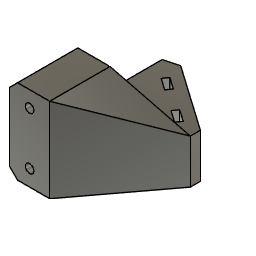
DirectDrive_SpoolHolder (Autodesk Fusion 360 design; units mm, degrees)
Autodesk Fusion 360 part; units mm, degrees
note: some values were not read from the file. Set by a fixed rule: which sketch regions a step uses.
sketch "Sketch1" plane through (0, 0, 0) normal (0, 0, 1) x (1, 0, 0) in component "Spool Holder"
  line L0 (10, 15) -> (-10, 15)
  line L1 (-10, 15) -> (-10, -15)
  line L2 (-10, -15) -> (10, -15)
  line L3 (10, -15) -> (10, 15)
  line L4 (10, 15) -> (-10, -15) construction
  line L5 (-10, 15) -> (10, -15) construction
  line L6 (10, 15) -> (50, 15)
  line L7 (50, 15) -> (50, 20)
  line L8 (50, 20) -> (17.2339, 42.9431)
  line L9 (50, 20) -> (46.0037, 20) construction
  line L10 (50, 15) -> (10, -15)
  line L11 (17.2339, 42.9431) -> (10, 32.612)
  line L12 (17.2339, 42.9431) -> (32.2339, 42.9431) construction
  line L13 (10, 15) -> (10, 32.612)
  line L14 (10, 32.612) -> (10, 41)
  line L15 (10, 41) -> (17.2339, 42.9431)
  dimension "d1" = 30
  dimension "d2" = 20
  dimension "d3" = 40
  dimension "d4" = 5
  dimension "d5" = 145
  dimension "d6" = 40
  dimension "d7" = 125
  constraint perpendicular L0 L1
  constraint parallel L0 L2
  constraint parallel L1 L3
  constraint horizontal L0
  constraint coincident L4 origin
  constraint coincident L5 origin
  constraint perpendicular L3 L6
  constraint perpendicular L6 L7
  constraint horizontal L9
  constraint horizontal L12
  constraint perpendicular L6 L13
  constraint vertical L14
  measures "d1" distance of L0.end L1.end
  measures "d2" distance of L1.end L2.end
  measures "d3" distance of L0.start L6.end
  measures "d4" distance of L6.end L7.end
  measures "d5" angle of L8 L9
  measures "d6" distance of L7.end L8.end
  measures "d7" angle of L11 L12
extrude "Extrude1" add sketch "Sketch1" along normal blind 42 in component "Spool Holder"
sketch "Sketch2" plane through (0, 0, 42) normal (0, 0, 1) x (-1, 0, 0) in component "Spool Holder"
  line L0 (10, -15) -> (10, 15)
  line L1 (10, 15) -> (-10, 15)
  line L2 (-10, 15) -> (-50, -15)
  line L3 (-50, -15) -> (-50, -20)
  line L4 (-50, -20) -> (-17.2339, -42.9431)
  line L5 (-10, -41) -> (-10, -15)
  line L6 (-10, -15) -> (10, -15)
  line L7 (-10, -15) -> (-50, -15)
  line L8 (-17.2339, -42.9431) -> (-10, -41)
  constraint coincident L5.end L6.start
  constraint coincident L2.end L3.start
extrude "Extrude2" cut sketch "Sketch2" against normal blind 10 contours L3 L4 L5 L7 L8 in component "Spool Holder"
sketch "Sketch3" plane through (0, 0, 0) normal (0, 0, -1) x (1, 0, 0) in component "Spool Holder"
  line L0 (-10, 15) -> (-10, -15)
  line L1 (-10, -15) -> (10, -15)
  line L2 (10, -15) -> (10, -41)
  line L3 (17.2339, -42.9431) -> (50, -20)
  line L4 (50, -20) -> (50, -15)
  line L5 (50, -15) -> (10, 15)
  line L6 (10, 15) -> (-10, 15)
  line L7 (10, -15) -> (50, -15)
  line L8 (10, -41) -> (17.2339, -42.9431)
  constraint coincident L1.end L2.start
  constraint coincident L4.end L5.start
extrude "Extrude3" cut sketch "Sketch3" against normal blind 10 contours L2 L3 L4 L7 L8 in component "Spool Holder"
sketch "Sketch4" plane through (0, 15, 0) normal (0, 1, 0) x (-1, 0, 0) in component "Spool Holder"
  line L0 (-50, 0) -> (10, 0)
  line L1 (10, 0) -> (10, 42)
  line L2 (10, 42) -> (-50, 42)
  line L3 (-50, 42) -> (-50, 32)
  line L4 (-50, 32) -> (-10, 32)
  line L5 (-10, 32) -> (-10, 10)
  line L6 (-10, 10) -> (-50, 10)
  line L7 (-50, 10) -> (-50, 0)
  line L8 (-10, 32) -> (-10, 42)
  line L9 (-10, 10) -> (-10, 0)
  line L10 (-10, 42) -> (-50, 32)
  line L11 (-10, 0) -> (-50, 10)
  point P0 (-10, 0)
  constraint coincident L4.end L5.start
  constraint coincident L2 L8.end
  constraint perpendicular L2 L8
  constraint coincident L5.end L6.start
  constraint coincident L0 P0
  constraint perpendicular L0 L9
  constraint coincident L3.end L4.start
  constraint coincident L6.end L7.start
extrude "Extrude4" cut sketch "Sketch4" along normal up to surface contours L0 L7 L11 | L2 L3 L10 end surface through (50, 15, 0) normal (0.6, -0.8, 0) offset 0 in component "Spool Holder"
sketch "Sketch5" plane through (0, 0, 32) normal (0, 0, 1) x (-1, 0, 0) in component "Spool Holder"
  line L0 (-10, -15) -> (-50, -15)
  line L1 (-50, -15) -> (-50, -20)
  line L2 (-50, -20) -> (-17.2339, -42.9431)
  line L3 (-10, -41) -> (-10, -15)
  line L4 (-17.2339, -42.9431) -> (-14.366, -38.8473) construction
  line L5 (-14.366, -38.8473) -> (-54.355, -10.8467) construction
  line L6 (-14.366, -38.8473) -> (-12.5879, -36.3079) construction
  line L7 (-12.5879, -36.3079) -> (-56.8094, -5.3437) construction
  line L8 (-50, -20) -> (-45.354, -13.3649) construction
  line L9 (-50, -20) -> (-58.1, -20) construction
  line L10 (-14.366, -38.8473) -> (-22.5576, -33.1115) construction
  line L11 (-22.5576, -33.1115) -> (-20.7795, -30.5722) construction
  line L12 (-47.1321, -15.9042) -> (-38.9406, -21.64) construction
  line L13 (-38.9406, -21.64) -> (-37.1625, -19.1006) construction
  line L14 (-22.5576, -33.1115) -> (-25.4655, -31.0753)
  line L15 (-25.4655, -31.0753) -> (-23.6875, -28.536)
  line L16 (-22.5576, -33.1115) -> (-19.6496, -35.1477)
  line L17 (-19.6496, -35.1477) -> (-17.8715, -32.6084)
  line L18 (-23.6875, -28.536) -> (-17.8715, -32.6084)
  line L19 (-38.9406, -21.64) -> (-41.8486, -19.6038)
  line L20 (-41.8486, -19.6038) -> (-40.0705, -17.0644)
  line L21 (-38.9406, -21.64) -> (-36.0326, -23.6762)
  line L22 (-36.0326, -23.6762) -> (-34.2545, -21.1368)
  line L23 (-40.0705, -17.0644) -> (-34.2545, -21.1368)
  line L24 (-17.2339, -42.9431) -> (-10, -41)
  dimension "d17" = 5
  dimension "d18" = 3.1
  dimension "d19" = 125
  dimension "d20" = 8.1
  dimension "d21" = 10
  dimension "d22" = 10
  dimension "d23" = 3.55
  dimension "d24" = 3.55
  dimension "d25" = 3.55
  dimension "d26" = 3.55
  constraint coincident L2.end L4.start
  constraint perpendicular L2 L4
  constraint perpendicular L5 L6
  constraint horizontal L9
  constraint coincident L1.end L2.start
  constraint perpendicular L6 L10
  constraint coincident L7 L11.end
  constraint perpendicular L7 L11
  constraint coincident L5 L12.start
  constraint coincident L8 L12.start
  constraint perpendicular L8 L12
  constraint coincident L7 L13.end
  constraint perpendicular L7 L13
  constraint perpendicular L11 L14
  constraint coincident L7 L15.end
  constraint perpendicular L7 L15
  constraint perpendicular L11 L16
  constraint coincident L7 L17.end
  constraint perpendicular L7 L17
  constraint perpendicular L13 L19
  constraint coincident L7 L20.end
  constraint perpendicular L7 L20
  constraint perpendicular L13 L21
  constraint coincident L7 L22.end
  constraint perpendicular L7 L22
  measures "d17" distance of L2.end L4.end
  measures "d18" distance of L4.end L6.end
  measures "d19" angle of L8 L9
  measures "d20" distance of L1.end L8.end
  measures "d21" distance of L4.end L10.end
  measures "d22" distance of L12.start L12.end
  measures "d23" distance of L10.end L14.end
  measures "d24" distance of L10.end L16.end
  measures "d25" distance of L12.end L19.end
  measures "d26" distance of L12.end L21.end
extrude "Extrude5" cut sketch "Sketch5" against normal up to surface (22 mm away) contours L14 L15 L16 L17 L18 | L19 L20 L21 L22 L23 in component "Spool Holder"
sketch "Sketch6" plane through (25.8464, 36.9125, 0) normal (0.573576, 0.819152, 0) x (-0.819152, 0.573576, 0) in component "Spool Holder"
  line L0 (-29.4861, 10) -> (10.5139, 10)
  line L1 (10.5139, 32) -> (-29.4861, 32)
  line L2 (-29.4861, 32) -> (-29.4861, 10)
  line L3 (10.5139, 10) -> (10.5139, 32) construction
  line L4 (10.5139, 21) -> (-29.4861, 21) construction
  line L5 (10.5139, 21) -> (0.5139, 21) construction
  line L6 (-29.4861, 21) -> (-19.4861, 21) construction
  circle A0 centre (0.5139, 21) radius 2
  circle A1 centre (-19.4861, 21) radius 2
  line L7 (10.5139, 10) -> (10.5139, 32)
  dimension "d29" = 10
  dimension "d30" = 10
  dimension "d31" = 4
  dimension "d32" = 4
  constraint coincident L0.end L3.start
  constraint coincident L1.start L3.end
  constraint midpoint L3 L4.start
  constraint midpoint L2 L4.end
  constraint perpendicular L3 L5
  constraint perpendicular L2 L6
  constraint coincident L5.end A0.centre
  constraint coincident L6.end A1.centre
  measures "d29" distance of L4.start L5.end
  measures "d30" distance of L4.end L6.end
  measures "d31" diameter of A0
  measures "d32" diameter of A1
extrude "Extrude6" cut sketch "Sketch6" against normal blind 11 contours A0 | A1 in component "Spool Holder"
sketch "Sketch7" plane through (0, 15, 0) normal (0, 1, 0) x (-1, 0, 0) in component "Spool Holder"
  line L0 (-10, 42) -> (-50, 32)
  line L1 (-50, 32) -> (-10, 32)
  line L2 (-10, 32) -> (-10, 10)
  line L3 (-10, 10) -> (-50, 10)
  line L4 (-50, 10) -> (-10, 0)
  line L5 (-10, 0) -> (10, 0)
  line L6 (10, 0) -> (10, 42)
  line L7 (10, 42) -> (-10, 42)
  line L8 (-10, 42) -> (-10, 0) construction
  line L9 (-10, 42) -> (10, 42) construction
  line L10 (0, 42) -> (0, 0) construction
  line L11 (0, 42) -> (0, 34) construction
  line L12 (0, 0) -> (0, 8) construction
  circle A0 centre (0, 34) radius 3.6
  circle A1 centre (0, 8) radius 3.6
  dimension "d35" = 8
  dimension "d36" = 8
  dimension "d37" = 7.2
  dimension "d38" = 7.2
  constraint coincident L0.start L7.end
  constraint coincident L4.end L5.start
  constraint coincident L6.end L7.start
  constraint midpoint L9 L10.start
  constraint coincident L10.end L12.start
  constraint perpendicular L7 L11
  constraint perpendicular L5 L12
  constraint coincident L11.end A0.centre
  constraint coincident L12.end A1.centre
  measures "d35" distance of L10.start L11.end
  measures "d36" distance of L10.end L12.end
  measures "d37" diameter of A0
  measures "d38" diameter of A1
extrude "Extrude7" cut sketch "Sketch7" against normal blind 4.8 contours A0 | A1 in component "Spool Holder"
sketch "Sketch8" plane through (0, 15, 0) normal (0, 1, 0) x (-1, 0, 0) in component "Spool Holder"
  circle A0 centre (0, 8) radius 3.6
  circle A1 centre (0, 34) radius 3.6
  line L0 (-10, 42) -> (-50, 32)
  line L1 (-50, 32) -> (-10, 32)
  line L2 (-10, 32) -> (-10, 10)
  line L3 (-10, 10) -> (-50, 10)
  line L4 (-50, 10) -> (-10, 0)
  line L5 (-10, 0) -> (10, 0)
  line L6 (10, 0) -> (10, 42)
  line L7 (10, 42) -> (-10, 42)
  circle A2 centre (0, 8) radius 2.15
  circle A3 centre (0, 34) radius 2.15
  dimension "d41" = 4.3
  dimension "d42" = 4.3
  constraint concentric A0 A2
  constraint concentric A1 A3
  measures "d41" diameter of A2
  measures "d42" diameter of A3
extrude "Extrude8" cut sketch "Sketch8" against normal up to surface (30 mm away) contours A2 | A3 in component "Spool Holder"
chamfer "Chamfer1" distance 4 angle 45 2 edges at (-10, 0, 0) (-10, 0, 42) in component "Spool Holder"
chamfer "Chamfer2" distance 3 angle 45 1 edges at (10, 15, 21) in component "Spool Holder"
component "Spool Holder" placed x (1, 0, 0) y (0, 1, 0) z (0, 0, 1) at (0, 0, 0)
equation "d23 = ( 7.1 / 2 ) * 1 mm"
equation "d24 = ( 7.1 / 2 ) * 1 mm"
equation "d25 = ( 7.1 / 2 ) * 1 mm"
equation "d26 = ( 7.1 / 2 ) * 1 mm"
